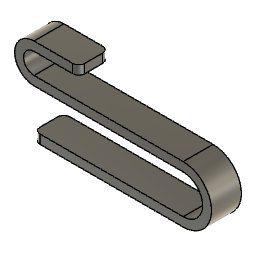
hookv2 v2 (Autodesk Fusion 360 design; units mm, degrees)
Autodesk Fusion 360 part; units mm, degrees
sketch "Sketch1" plane through (0, 0, 0) normal (0, 1, 0) x (1, 0, 0)
  line L0 (0, 0) -> (50, 0)
  line L1 (50, 3) -> (0, 3)
  line L2 (0, 3) -> (0, 0)
  line L3 (50, -13) -> (0, -13)
  line L4 (0, -16) -> (50, -16)
  line L5 (0, -23) -> (15, -23)
  line L6 (15, -23) -> (15, -26)
  line L7 (15, -26) -> (0, -26)
  arc A0 (0, -13) -> (0, -26) centre (0, -19.5) ccw
  arc A1 (0, -16) -> (0, -23) centre (0, -19.5) ccw
  arc A2 (50, -16) -> (50, 3) centre (50, -6.5) ccw
  arc A3 (50, -13) -> (50, 0) centre (50, -6.5) ccw
  constraint horizontal L0
  constraint horizontal L1
  constraint vertical L2
  constraint coincident L0.start L2.end
  constraint horizontal L3
  constraint horizontal L4
  constraint horizontal L5
  constraint vertical L6
  constraint horizontal L7
  constraint tangent L5 A1
  constraint tangent L7 A0
  constraint tangent L3 A3
  constraint tangent L4 A2
extrude "Extrude1" add sketch "Sketch1" along normal blind 10
fillet "Fillet1" radius 2 1 edges at (15, 0, 24.5)
fillet "Fillet2" radius 2 1 edges at (15, 10, 24.5)
fillet "Fillet3" radius 2 1 edges at (0, 0, -1.5)
fillet "Fillet4" radius 2 1 edges at (0, 10, -1.5)
